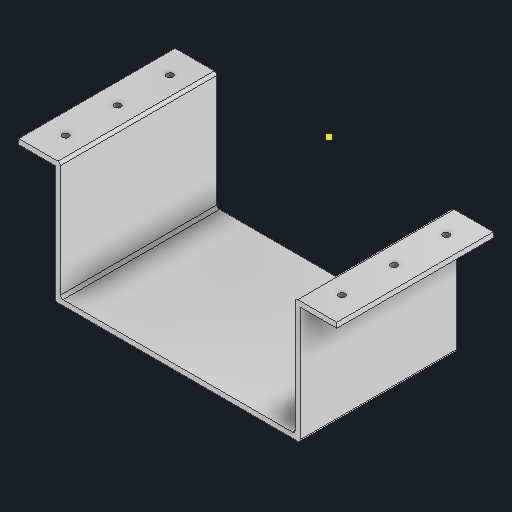
# Autodesk Inventor part: Top joint housing back
Saved by Autodesk Inventor 2026.3 (Build 303398000, 398)
## iProperties
Created: 2026-07-26
Part Number: Top joint housing back
Material: Generic
Document SubType Name: Sheet Metal
Designer: matot
Density: 1 g/cm^3
Sheet Metal Rule: Default_mm
Appearance: Default
Author: matot
Autodesk Inventor part; units mm, degrees
ref_plane "YZ Plane" through (0, 0, 0) normal (1, 0, 0) x (0, 1, 0)
ref_plane "XZ Plane" through (0, 0, 0) normal (0, 1, 0) x (-1, 0, 0)
ref_plane "XY Plane" through (0, 0, 0) normal (0, 0, 1) x (1, 0, 0)
sketch "Sketch1" plane through (0, 0, 0) normal (0, 0, 1) x (1, 0, 0)
  line L0 (98, 0) -> (98, -90)
  line L1 (98, -90) -> (-90, -90)
  line L2 (-90, -90) -> (-90, 0)
  line L3 (126, 4) -> (126, 0)
  line L4 (126, 0) -> (-118, 0)
  line L5 (-118, 0) -> (-118, 4)
  line L6 (-86, 4) -> (94, 4)
  line L7 (94, 4) -> (94, -86)
  line L8 (94, -86) -> (-86, -86)
  line L9 (-86, -86) -> (-86, 4)
  line L10 (-90, 0) -> (-86, 0)
  line L11 (94, 0) -> (98, 0)
  line L12 (-118, 4) -> (-86, 4)
  line L13 (94, 4) -> (126, 4)
  point P0 (0, 0)
  point P1 (6, -4)
  point P2 (126, 2)
  point P3 (98, 0)
  dimension "d0" = 188
  dimension "d1" = 90
  dimension "d3" = 90
  dimension "d4" = 244
  dimension "d5" = 120
  dimension "d8" = 90
  dimension "d9" = 180
  dimension "d10" = 4
  dimension "d13" = 0
  dimension "d14" = 4
  dimension "d91" = 32
  constraints: 28 end point, 8 parallel, 5 horizontal, 5 perpendicular, 2 point on line, 1 midpoint
  measures "d0" distance of L0.end L1.end
  measures "d1" distance of L0.start L0.end
  measures "d3" distance from line of point (0, 0) L2
  measures "d4" distance of L5.end L3.start
  measures "d5" horizontal distance of point (6, -4) point (126, 2)
  measures "d8" distance of L6.end L7.end
  measures "d9" distance of L7.end L8.end
  measures "d10" distance between parallel lines of L0 L7
  measures "d13" distance from line of point (0, 0) L4
  measures "d14" distance between parallel lines of L4 L12
  measures "d91" distance from line of L7 point (126, 2)
extrude "Extrusion1" add sketch "Sketch1" along normal blind 120 contours L4 L7 L13 L3 | L0 L1 L2 L4 L9 L8 L7 | L4 L5 L12 L9
fillet "Fillet1" radius 2 4 edges at (-86, -86, 60) (-86, 4, 60) (94, 4, 60) (98, -90, 60)
fillet "Fillet2" radius 2 2 edges at (-90, -90, 60) (94, -86, 60)
sketch "Sketch7" plane through (-118, 4, 120) normal (0, 1, 0) x (1, 0, 0)
  point P0 (118, 120)
sketch "Sketch8" plane through (126, 4, 120) normal (0, 1, 0) x (1, 0, 0)
  line L0 (0, 120) -> (0, 0) projected
  line L1 (-34, 0) -> (-210, 0) projected
  line L2 (-244, 120) -> (-244, 0) projected
  line L3 (-214, 0) -> (-244, 0) projected
  point P0 (-126, 120)
  point P1 (-16, 100)
  point P2 (-16, 60)
  point P3 (-16, 20)
  point P4 (-228, 100)
  point P5 (-228, 60)
  point P6 (-228, 20)
  dimension "d72" = 16
  dimension "d73" = 16
  dimension "d74" = 16
  dimension "d75" = 20
  dimension "d76" = 40
  dimension "d77" = 40
  dimension "d78" = 16
  dimension "d79" = 40
  dimension "d80" = 40
  dimension "d81" = 20
  dimension "d82" = 16
  dimension "d83" = 16
  measures "d72" distance from line of point (-16, 20) L0
  measures "d73" distance from line of point (-16, 60) L0
  measures "d74" distance from line of point (-16, 100) L0
  measures "d75" distance from line of L1 point (-16, 20)
  measures "d76" distance of point (-16, 60) point (-16, 20)
  measures "d77" distance of point (-16, 100) point (-16, 60)
  measures "d78" distance from line of L2 point (-228, 20)
  measures "d79" distance of point (-228, 20) point (-228, 60)
  measures "d80" distance of point (-228, 60) point (-228, 100)
  measures "d81" distance from line of point (-228, 20) L3
  measures "d82" distance from line of L2 point (-228, 60)
  measures "d83" distance from line of point (-228, 100) L2
hole "Hole6" at (110, 4, 20) at (110, 4, 60) at (110, 4, 100) at (-102, 4, 20) at (-102, 4, 60) at (-102, 4, 100) direction (0, -1, 0) diameter 4.917 end through all thread size "M6x1" class "6H" standard "ISO Metric profile"
equation "\"d89\" = Thickness"
equation "\"BendRadius\" = Thickness"
equation "\"BendReliefWidth\" = Thickness"
equation "\"BendReliefDepth\" = 0.5 * Thickness"
equation "\"CornerReliefSize\" = 4 * Thickness"
equation "\"MinimumRemnant\" = 2 * Thickness"
equation "\"TransitionRadius\" = BendRadius"
equation "\"JacobiRadiusSize\" = BendRadius"
equation "\"GapSize\" = Thickness"
equation "\"Thickness\" = 0.5"
body "Solid1"
